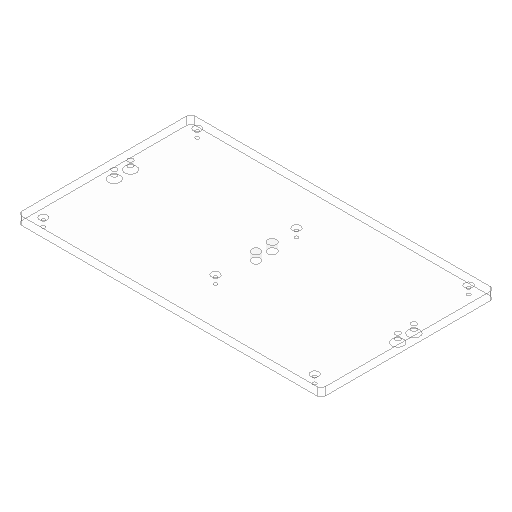
# Autodesk Inventor part: FCT-01-171A
Saved by Autodesk Inventor 2026.1 (Build 301233000, 233)
## iProperties
Company: Delta
Created: 2025-08-15
Part Number: FCT-01-171A
Material: Acrílico TP
Document SubType Name: Modeling
Designer: Willian Pinheiro
Density: 1.19 g/cm^3
Appearance: Transparente - Claro
Project: FCT
Description: Base Pressor 1
Mass: 948.252 g
Surface Area: 1734.87 cm^2
Volume: 796.85 cm^3
Checked By: Antonio Lucas
Engr Approved By: Antonio Lucas
Mfg Approved By: Anderson Oliveira
Acabamento: N/A
Dimensões: 10 x 214 x 375
Total: 1
Author: Willian Pinheiro
Revision Number: 01
Title: FCT
Autodesk Inventor part; units mm, degrees
ref_plane "YZ Plane" through (0, 0, 0) normal (1, 0, 0) x (0, 1, 0)
ref_plane "XZ Plane" through (0, 0, 0) normal (0, 1, 0) x (-1, 0, 0)
ref_plane "XY Plane" through (0, 0, 0) normal (0, 0, 1) x (1, 0, 0)
sketch "Sketch1" plane through (0, 0, 0) normal (0, 0, 1) x (1, 0, 0)
  line L0 (-262.5, 0) -> (262.5, 0) construction
  line L1 (0, -149.8) -> (0, 149.8) construction
  line L2 (-187.5, 107) -> (187.5, 107)
  line L3 (187.5, 107) -> (187.5, -107)
  line L4 (187.5, -107) -> (-187.5, -107)
  line L5 (-187.5, -107) -> (-187.5, 107)
  point P0 (-167.5, 95)
  point P1 (167.5, 95)
  point P2 (-167.5, -95)
  point P3 (167.5, -95)
  point P4 (0, 0)
  point P5 (-175, 0)
  point P6 (175, 0)
  point P7 (0, -50)
  point P8 (0, 50)
  point P9 (0, 20)
  point P10 (175, 20)
  point P11 (-175, 20)
  dimension "d0" = 375
  dimension "d1" = 214
  dimension "d3" = 335
  dimension "d30" = 20
  dimension "d45" = 12
  dimension "d46" = 190
  dimension "d47" = 100
  dimension "d48" = 12.5
  dimension "d52" = 20
  constraints: 8 end point, 6 symmetric about line, 5 point on line, 2 horizontal alignment, 2 midpoint, 2 parallel, 1 horizontal, 1 perpendicular, 1 vertical alignment, 2 other
  measures "d0" distance between parallel lines of L3 L5
  measures "d1" distance between parallel lines of L4 L2
  measures "d3" distance of point (167.5, 95) point (-167.5, 95)
  measures "d30" distance from line of L5 point (-167.5, 95)
  measures "d45" distance from line of L2 point (-167.5, 95)
  measures "d46" distance of point (-167.5, -95) point (-167.5, 95)
  measures "d47" distance of point (0, -50) point (0, 50)
  measures "d48" distance from line of L5 point (-175, 0)
  measures "d52" distance of point (-175, 20) point (-175, 0)
extrude "Extrusion1" add sketch "Sketch1" against normal blind 10
hole "Hole1" at (-167.5, 95, 0) at (167.5, 95, 0) at (-167.5, -95, 0) at (167.5, -95, 0) at (0, -50, 0) at (0, 50, 0) direction (0, 0, -1) diameter 4.5 end through all countersink diameter 10 countersink angle 90 clearance for "Countersunk Flat Head Hex Socket Screw ISO 10642" size "M4" standard "ISO"
hole "Hole2" at (0, 0, 0) at (0, 20, 0) direction (0, 0, -1) diameter 10.647 end through all thread size "M12x1.25" class "6H" standard "ISO Metric profile"
sketch "Sketch2" plane through (0, 0, -10) normal (0, 0, -1) x (-1, 0, 0)
  point P0 (0, 0)
  point P1 (175, 0)
  point P2 (175, 0)
  point P3 (-175, 0)
  point P4 (-175, 0)
  point P5 (0, 20)
  point P6 (0, 0)
  point P7 (175, 20)
  point P8 (-175, 20)
  constraints: 2 coincident
hole "Hole4" at (-175, 0, -10) at (175, 0, -10) at (-175, 20, -10) at (175, 20, -10) direction (0, 0, 1) diameter 6.5 end through all countersink diameter 14.5 countersink angle 90 clearance for "Countersunk Flat Head Hex Socket Screw ISO 10642" size "M6" standard "ISO"
fillet "Arredondamento2" radius 5 4 edges at (187.5, -107, -5) (187.5, 107, -5) (-187.5, -107, -5) (-187.5, 107, -5)
body "Solid1"
